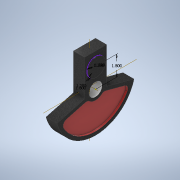
# Autodesk Inventor part: crankshaft counterwieght
Saved by Autodesk Inventor 2021.1 (Build 251245000, 245)
## iProperties
Created: 2020-08-31
Part Number: crankshaft counterwieght
Material: Generic
Document SubType Name: Sheet Metal
Designer: Vamshi
Density: 1 g/cm^3
Sheet Metal Rule: Default
Appearance: Default
Author: Vamshi
Autodesk Inventor part; units mm, degrees
ref_plane "YZ Plane" through (0, 0, 0) normal (1, 0, 0) x (0, 1, 0)
ref_plane "XZ Plane" through (0, 0, 0) normal (0, 1, 0) x (-1, 0, 0)
ref_plane "XY Plane" through (0, 0, 0) normal (0, 0, 1) x (1, 0, 0)
sketch "Sketch1" plane through (0, 0, 0) normal (0, 0, 1) x (1, 0, 0)
  arc A0 (-88.3243, -23.6664) -> (88.3243, -23.6664) centre (0, 0) ccw
  line L0 (-25.4, 76.2) -> (25.4, 76.2)
  line L1 (25.4, 76.2) -> (25.4, -6.8059)
  line L2 (-25.4, -6.8059) -> (-25.4, 76.2)
  line L3 (-25.4, -6.8059) -> (-88.3243, -23.6664)
  line L4 (25.4, -6.8059) -> (88.3243, -23.6664)
  line L5 (0, -124.968) -> (0, 109.728) projected
  constraints: 10 end point, 2 point on circle, 1 centre point, 1 coincident, 1 horizontal, 1 parallel, 1 perpendicular, 1 other
extrude "Extrusion1" add sketch "Sketch1" against normal mid plane 25.4
sketch "Sketch2" plane through (0, 0, -12.7) normal (0, 0, -1) x (-1, 0, 0)
  circle A0 centre (0, 0) radius 15.24
  circle A1 centre (0, 0) radius 20.32
  dimension "d7" = 30.48
  dimension "d8" = 40.64
  constraints: 2 centre point, 2 coincident
  measures "d7" diameter of A0
  measures "d8" diameter of A1
extrude "Extrusion2" cut sketch "Sketch2" against normal through all contours A0
extrude "Extrusion3" add sketch "Sketch2" along normal blind 2.54 contours A0 | A1
sketch "Sketch3" plane through (0, 0, 12.7) normal (0, 0, 1) x (1, 0, 0)
  circle A0 centre (0, 45.72) radius 15.24
  circle A1 centre (0, 45.72) radius 20.32
  point P0 (0, 0)
  dimension "d13" = 30.48
  dimension "d14" = 40.64
  dimension "d15" = 45.72
  constraints: 2 centre point, 1 coincident
  measures "d13" diameter of A0
  measures "d14" diameter of A1
  measures "d15" distance of point (0, 0) A0.centre
extrude "Extrusion4" cut sketch "Sketch3" against normal through all contours A0
extrude "Extrusion5" add sketch "Sketch3" along normal blind 2.54 contours A0 | A1
sketch "Sketch4" plane through (0, 0, 12.7) normal (0, 0, 1) x (1, 0, 0)
  arc A0 (-73.3333, -40.5957) -> (73.3333, -40.5957) centre (0, 0) ccw
  circle A1 centre (0, 45.72) radius 20.32 projected
  circle A2 centre (0, 45.72) radius 15.24 projected
  circle A3 centre (0, 0) radius 15.24 projected
  line L0 (25.4, -6.8059) -> (88.3243, -23.6664) projected
  arc A4 (-88.3243, -23.6664) -> (88.3243, -23.6664) centre (0, 0) ccw projected
  line L1 (-88.3243, -23.6664) -> (-25.4, -6.8059) projected
  line L2 (-25.4, -6.8059) -> (-25.4, 76.2) projected
  line L3 (-25.4, 76.2) -> (25.4, 76.2) projected
  line L4 (25.4, 76.2) -> (25.4, -6.8059) projected
  circle A5 centre (0, 45.72) radius 20.32 projected
  circle A6 centre (0, 0) radius 15.24 projected
  arc A7 (-88.3243, -23.6664) -> (88.3243, -23.6664) centre (0, 0) ccw projected
  line L5 (88.3243, -23.6664) -> (25.4, -6.8059) projected
  line L6 (25.4, -6.8059) -> (25.4, 76.2) projected
  line L7 (25.4, 76.2) -> (-25.4, 76.2) projected
  line L8 (-25.4, 76.2) -> (-25.4, -6.8059) projected
  line L9 (-25.4, -6.8059) -> (-88.3243, -23.6664) projected
  line L10 (-67.074, -25.8612) -> (-23.4361, -14.1685)
  line L11 (23.4361, -14.1685) -> (67.074, -25.8612)
  arc A8 (-67.074, -25.8612) -> (-73.3333, -40.5957) centre (-64.4444, -35.675) ccw
  arc A9 (73.3333, -40.5957) -> (67.074, -25.8612) centre (64.4444, -35.675) ccw
  arc A10 (-14.1484, -16.308) -> (14.1484, -16.308) centre (0, 0) ccw
  arc A11 (-14.1484, -16.308) -> (-23.4361, -14.1685) centre (-20.8065, -23.9823) ccw
  arc A12 (23.4361, -14.1685) -> (14.1484, -16.308) centre (20.8065, -23.9823) ccw
  point P0 (78.6564, -28.9647)
  point P1 (-78.6564, -28.9647)
  point P2 (-17.5401, -12.5887)
  point P3 (17.5401, -12.5887)
  dimension "d20" = 167.64
  dimension "d21" = 7.62
  dimension "d22" = 7.62
  dimension "d23" = 10.16
  dimension "d24" = 43.18
  dimension "d25" = 10.16
  constraints: 16 point on circle, 8 tangent, 6 centre point, 4 end point, 4 point on line, 2 coincident, 2 equal radius, 2 parallel
  measures "d20" diameter of A0
  measures "d21" distance between parallel lines of L10 L1
  measures "d22" distance between parallel lines of L0 L11
  measures "d23" radius of A8
  measures "d24" diameter of A10
  measures "d25" radius of A11
extrude "Extrusion6" cut sketch "Sketch4" against normal blind 5.08 contours A8 L10 A11 A10 A12 L11 A9 A0
mirror "Mirror1" about plane through (0, 0, 0) normal (0, 0, 1) of "Extrusion6"
equation "\"BendRadius\" = Thickness"
equation "\"BendReliefWidth\" = Thickness"
equation "\"BendReliefDepth\" = 0.5 * Thickness"
equation "\"CornerReliefSize\" = 4 * Thickness"
equation "\"MinimumRemnant\" = 2 * Thickness"
equation "\"TransitionRadius\" = BendRadius"
equation "\"JacobiRadiusSize\" = BendRadius"
equation "\"GapSize\" = Thickness"
equation "\"Thickness\" = 3.048"
body "Solid1"
